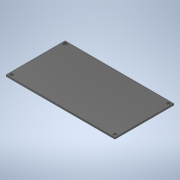
# Autodesk Inventor part: MainBoard
Saved by Autodesk Inventor 2020.4 (Build 244396000, 396)
## iProperties
Part Number: MainBoard
Material: 一般
Document SubType Name: Modeling
Designer: Masato Kubotera
Density: 1 g/cm^3
Appearance: 滑らか - 黒
Mass: 13.3885 g
Surface Area: 174.08 cm^2
Volume: 13.3885 cm^3
Description: CircuitBoard
Author: Masato Kubotera
Autodesk Inventor part; units mm, degrees
ref_plane "YZ Plane" through (0, 0, 0) normal (1, 0, 0) x (0, 1, 0)
ref_plane "XZ Plane" through (0, 0, 0) normal (0, 1, 0) x (-1, 0, 0)
ref_plane "XY Plane" through (0, 0, 0) normal (0, 0, 1) x (1, 0, 0)
sketch "スケッチ1" plane through (0, 0, 0) normal (0, 0, 1) x (1, 0, 0)
  line L0 (32.5, 60) -> (-32.5, 60)
  line L1 (-32.5, 60) -> (-32.5, -60)
  line L2 (-32.5, -60) -> (32.5, -60)
  line L3 (32.5, -60) -> (32.5, 60)
  line L4 (32.5, 60) -> (-32.5, -60) construction
  line L5 (-32.5, 60) -> (32.5, -60) construction
  line L6 (32.5, 0) -> (-32.5, 0) construction
  line L7 (0, 60) -> (0, -60) construction
  circle A0 centre (29.5, 57) radius 1.6
  line L8 (-29.5, -57) -> (29.5, -57) construction
  line L9 (29.5, -57) -> (29.5, 57) construction
  line L10 (29.5, 57) -> (-29.5, 57) construction
  line L11 (-29.5, 57) -> (-29.5, -57) construction
  line L12 (-29.5, -57) -> (29.5, 57) construction
  line L13 (29.5, -57) -> (-29.5, 57) construction
  circle A1 centre (29.5, -57) radius 1.6
  circle A2 centre (-29.5, 57) radius 1.6
  circle A3 centre (-29.5, -57) radius 1.6
  point P0 (0, 0)
  dimension "d0" = 65
  dimension "d1" = 120
  dimension "d2" = 3.2
  dimension "d3" = 59
  dimension "d4" = 114
  constraints: 28 end point, 8 midpoint, 4 centre point, 4 parallel, 3 symmetric about line, 2 horizontal, 2 perpendicular, 1 coincident, 3 other
  measures "d0" distance of L2.end L1.end
  measures "d1" distance of L1.end L0.end
  measures "d2" diameter of A0
  measures "d3" distance of L10.end L9.end
  measures "d4" distance of L9.end L8.end
extrude "押し出し1" add sketch "スケッチ1" along normal blind 1.6
